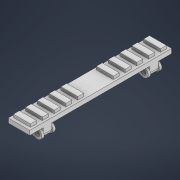
# Autodesk Inventor part: McCrea_CHAIN_INK_WALLE
Saved by Autodesk Inventor 2022 (Build 260153000, 153)
## iProperties
Created: 2021-12-29
Part Number: McCrea_CHAIN_INK_WALLE
Material: Generic
Document SubType Name: Modeling
Designer: MatusBarany
Density: 1 g/cm^3
Appearance: Default
Author: MatusBarany
Autodesk Inventor part; units mm, degrees
ref_plane "YZ Plane" through (0, 0, 0) normal (1, 0, 0) x (0, 1, 0)
sketch "Sketch2" plane through (0, 0, 0) normal (0, 0, 1) x (1, 0, 0)
  circle A0 centre (2.5, 0) radius 1.5
  circle A1 centre (-2.5, 0) radius 1.5
  arc A2 (-1.9231, 1.3846) -> (1.9231, 1.3846) centre (0, 6) ccw
  arc A3 (1.9231, -1.3846) -> (-1.9231, -1.3846) centre (0, -6) ccw
  circle A4 centre (2.5, 0) radius 0.75
  circle A5 centre (-2.5, 0) radius 0.75
  point P0 (0, 0)
  dimension "d0" = 3
  dimension "d1" = 3
  dimension "d2" = 6
  dimension "d3" = 6
  dimension "d4" = 2.5
  dimension "d5" = 2.5
  dimension "d6" = 1.5
  dimension "d7" = 1.5
  constraints: 8 point on circle, 6 centre point, 4 tangent, 2 coincident, 2 horizontal alignment
  measures "d0" diameter of A1
  measures "d1" diameter of A0
  measures "d2" distance of A2.centre point (0, 0)
  measures "d3" distance of point (0, 0) A3.centre
  measures "d4" distance of point (0, 0) A0.centre
  measures "d5" distance of A1.centre point (0, 0)
  measures "d6" diameter of A5
  measures "d7" diameter of A4
extrude "Extrusion2" add sketch "Sketch2" along normal blind 0.8
sketch "Sketch3" plane through (0, 0, 0) normal (0, 0, -1) x (-1, 0, 0)
  arc A0 (1.9231, -1.3846) -> (-1.9231, -1.3846) centre (0, -6) ccw projected
  arc A1 (1.9231, -1.3846) -> (1.9231, 1.3846) centre (2.5, 0) ccw projected
  arc A2 (-1.9231, 1.3846) -> (1.9231, 1.3846) centre (0, 6) ccw projected
  arc A3 (-1.9231, 1.3846) -> (-1.9231, -1.3846) centre (-2.5, 0) ccw projected
  circle A4 centre (-2.5, 0) radius 0.75 projected
  circle A5 centre (2.5, 0) radius 0.75 projected
  circle A6 centre (-2.5, 0) radius 1.125
  line L0 (-3.625, 2) -> (-1.375, 2)
  line L1 (-1.375, 2) -> (-1.375, 0)
  line L2 (-3.625, 0) -> (-3.625, 2)
  line L3 (0, -8.4) -> (0, 8.4) projected
  point P0 (0, 0)
  point P1 (-3.4922, 1.125)
  point P2 (-3.625, 0.9922)
  point P3 (-1.375, 1.1928)
  dimension "d12" = 2.25
  dimension "d16" = 1.5
  dimension "d20" = 2
  constraints: 6 end point, 2 parallel, 2 point on circle, 2 tangent, 1 centre point, 1 coincident, 1 perpendicular
  measures "d12" diameter of A6
  measures "d16" radius of A3
  measures "d20" distance of L0.end L1.end
extrude "Extrusion3" add sketch "Sketch3" along normal blind 1.5 contours L2 L0 L1 A2 A3 | A3 A2 L1 A6 L2 | A6
mirror "Mirror1" about plane through (0, 0, 0) normal (1, 0, 0) of "Extrusion3"
ref_plane "Work Plane1" through (-2.5, 0, -1.5) normal (0, 0, -1) x (-1, 0, 0)
mirror "Mirror2" about plane through (-2.5, 0, -1.5) normal (0, 0, -1) of "Extrusion3", "Mirror1", "Extrusion2"
sketch "Sketch4" plane through (1.375, 2, 0) normal (0, 1, 0) x (1, 0, 0)
  line L0 (-5, -4.5) -> (2.25, -4.5)
  line L1 (2.25, -4.5) -> (2.25, 1.5)
  line L2 (-5, 1.5) -> (-5, -4.5)
  line L3 (-2.75, 0) -> (-5, 0) projected
  line L4 (-2.75, 0) -> (-2.75, 3) projected
  line L5 (-2.75, 3) -> (-5, 3) projected
  line L6 (-5, 0) -> (-5, 3) projected
  line L7 (0, 0) -> (2.25, 0) projected
  line L8 (2.25, 0) -> (2.25, 3) projected
  line L9 (0, 3) -> (2.25, 3) projected
  line L10 (0, 0) -> (0, 3) projected
  line L11 (-5, 0) -> (-5, 3) projected
  line L12 (2.25, 0) -> (2.25, 3) projected
  line L13 (2.25, 1.5) -> (-5, 1.5)
  line L14 (2.25, 1.5) -> (-5, 1.5)
  line L15 (-5, 1.5) -> (-5, 19.5)
  line L16 (-5, 19.5) -> (2.25, 19.5)
  line L17 (2.25, 19.5) -> (2.25, 1.5)
  point P0 (-1.375, 0)
  point P1 (2.25, 1.5)
  point P2 (2.25, 3)
  dimension "d22" = 18
  dimension "d23" = 6
  constraints: 16 end point, 3 parallel, 2 collinear, 2 horizontal, 2 midpoint, 2 perpendicular
  measures "d22" distance between parallel lines of L14 L16
  measures "d23" distance of L2.start L0.start
extrude "Extrusion4" add sketch "Sketch4" along normal blind 1.5
sketch "Sketch5" plane through (1.375, 3.5, 0) normal (0, 1, 0) x (1, 0, 0)
  line L0 (1.5, -1.5) -> (-4.25, -1.5)
  line L1 (-4.25, -1.5) -> (-4.25, -3.5)
  line L2 (-4.25, -3.5) -> (1.5, -3.5)
  line L3 (1.5, -3.5) -> (1.5, -1.5)
  line L4 (-5, -4.5) -> (2.25, -4.5) projected
  line L5 (2.25, -4.5) -> (2.25, 19.5) projected
  line L6 (2.25, 19.5) -> (-5, 19.5) projected
  line L7 (-5, 19.5) -> (-5, -4.5) projected
  point P0 (-1.375, 0)
  dimension "d26" = 5.75
  dimension "d27" = 7.25
  dimension "d28" = 2
  dimension "d29" = 0.75
  dimension "d30" = 1
  constraints: 8 end point, 2 parallel, 1 horizontal, 1 perpendicular
  measures "d26" distance of L1.end L2.end
  measures "d27" distance of L4.start L4.end
  measures "d28" distance of L0.end L1.end
  measures "d29" distance between parallel lines of L1 L7
  measures "d30" distance between parallel lines of L4 L2
extrude "Extrusion5" add sketch "Sketch5" along normal blind 1 contours L3 L2 L1 L0
pattern_linear "Rectangular Pattern1" count 5 spacing 4 along (0, 0, -1) of "Extrusion5"
ref_plane "Work Plane2" through (3.625, 2, -19.5) normal (0, 0, -1) x (-1, 0, 0)
mirror "Mirror3" about plane through (3.625, 2, -19.5) normal (0, 0, -1) of "Extrusion4", "Extrusion3", "Mirror1", "Extrusion2", "Mirror2", "Extrusion5", "Rectangular Pattern1"
equation "\"d1\" = d0"
equation "\"d2\" = 2 * d0"
equation "\"d3\" = d2"
equation "\"d4\" = d5"
equation "\"d7\" = d6"
equation "\"d12\" = d16 + 0.5 * d13"
equation "\"d29\" = -0.5 * d26 + 0.5 * d27"
equation "\"d13\" = 1.5"
body "Solid2"
